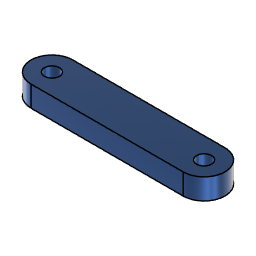
Servo Link v7 (Autodesk Fusion 360 design; units mm, degrees)
Autodesk Fusion 360 part; units mm, degrees
sketch "Sketch1" plane through (0, 0, 0) normal (0, 0, 1) x (1, 0, 0)
  line L0 (0, -2.5) -> (18.2, -2.5)
  arc A0 (18.2, -2.5) -> (18.2, 2.5) centre (18.2, 0) ccw
  line L1 (18.2, 2.5) -> (0, 2.5)
  arc A1 (0, 2.5) -> (0, -2.5) centre (0, 0) ccw
  line L2 (0, 0) -> (18.2, 0) construction
  circle A2 centre (0, 0) radius 0.9
  circle A3 centre (18.2, 0) radius 0.9
  dimension "d1" = 18.2
  dimension "d2" = 1.8
  dimension "d3" = 1.8
  dimension "d4" = 2.5
  constraint tangent L0 A0
  constraint tangent A0 L1
  constraint parallel L0 L1
  constraint tangent L1 A1
  constraint tangent L0 A1
  constraint horizontal L2
  constraint coincident A1.centre L2.start
  constraint concentric A0 A3
  measures "d1" distance of A1.centre A0.centre
  measures "d2" diameter of A2
  measures "d3" diameter of A3
  measures "d4" radius of A0
extrude "Extrude1" add sketch "Sketch1" along normal blind 2.5
